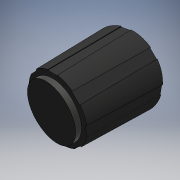
# Autodesk Inventor part: Knob-K60-S150
Saved by Autodesk Inventor 2018 (Build 220112000, 112)
## iProperties
Created: 2020-04-22
Part Number: Knob-K60-S150
Material: Všeobecné
Document SubType Name: Modeling
Designer: Jozko Mrkvicka
Density: 1 g/cm^3
Appearance: Výchozí
Author: Jozko Mrkvicka
Autodesk Inventor part; units mm, degrees
ref_plane "YZ Plane" through (0, 0, 0) normal (1, 0, 0) x (0, 1, 0)
ref_plane "XZ Plane" through (0, 0, 0) normal (0, 1, 0) x (-1, 0, 0)
ref_plane "XY Plane" through (0, 0, 0) normal (0, 0, 1) x (1, 0, 0)
sketch "Náčrt7" plane through (0, 0, 0) normal (0, 1, 0) x (-1, 0, 0)
  line L0 (7.4412, 0.9375) -> (7.3039, 0.9375)
  line L1 (7.3039, 0.9375) -> (7.3039, -0.9375)
  line L2 (7.3039, -0.9375) -> (7.4412, -0.9375)
  line L3 (-7.4412, -0.9375) -> (-7.3039, -0.9375)
  line L4 (-7.3039, -0.9375) -> (-7.3039, 0.9375)
  line L5 (-7.3039, 0.9375) -> (-7.4412, 0.9375)
  line L6 (-0.9375, 7.4412) -> (-0.9375, 7.3039)
  line L7 (-0.9375, 7.3039) -> (0.9375, 7.3039)
  line L8 (0.9375, 7.3039) -> (0.9375, 7.4412)
  line L9 (0.9375, -7.4412) -> (0.9375, -7.3039)
  line L10 (0.9375, -7.3039) -> (-0.9375, -7.3039)
  line L11 (-0.9375, -7.3039) -> (-0.9375, -7.4412)
  line L12 (-4.5988, -5.9246) -> (-4.5017, -5.8276)
  line L13 (-4.5017, -5.8276) -> (-5.8276, -4.5017)
  line L14 (-5.8276, -4.5017) -> (-5.9246, -4.5988)
  line L15 (4.5988, 5.9246) -> (4.5017, 5.8276)
  line L16 (4.5017, 5.8276) -> (5.8276, 4.5017)
  line L17 (5.8276, 4.5017) -> (5.9246, 4.5988)
  line L18 (5.9246, -4.5988) -> (5.8276, -4.5017)
  line L19 (5.8276, -4.5017) -> (4.5017, -5.8276)
  line L20 (4.5017, -5.8276) -> (4.6432, -5.969)
  line L21 (-5.9246, 4.5988) -> (-5.8276, 4.5017)
  line L22 (-5.8276, 4.5017) -> (-4.5017, 5.8276)
  line L23 (-4.5017, 5.8276) -> (-4.5988, 5.9246)
  arc A0 (5.9246, -4.5988) -> (7.4412, -0.9375) centre (0, 0) ccw
  arc A1 (0.9375, -7.4412) -> (4.5988, -5.9246) centre (0, 0) ccw
  arc A2 (-4.5988, -5.9246) -> (-0.9375, -7.4412) centre (0, 0) ccw
  arc A3 (-7.4412, -0.9375) -> (-5.9246, -4.5988) centre (0, 0) ccw
  arc A4 (-5.9246, 4.5988) -> (-7.4412, 0.9375) centre (0, 0) ccw
  arc A5 (-0.9375, 7.4412) -> (-4.5988, 5.9246) centre (0, 0) ccw
  arc A6 (7.4412, 0.9375) -> (5.9246, 4.5988) centre (0, 0) ccw
  arc A7 (4.5988, 5.9246) -> (0.9375, 7.4412) centre (0, 0) ccw
  point P0 (8, 0)
  point P1 (5.6569, -5.6569)
  point P2 (0, -8)
  point P3 (-5.6569, -5.6569)
  point P4 (-8, 0)
  point P5 (-5.6569, 5.6569)
  point P6 (0.0625, 7.5039)
  point P7 (5.6569, 5.6569)
  dimension "d237" = 0.2
  dimension "d239" = 7.5
  dimension "d240" = 7.5
  dimension "d241" = 7.5
  dimension "d242" = 7.5
  dimension "d243" = 7.5
  dimension "d244" = 7.5
  dimension "d245" = 7.5
  dimension "d246" = 7.5
  constraints: 48 end point, 16 point on circle, 8 centre point, 8 parallel, 8 perpendicular, 1 coincident, 1 horizontal, 1 point on line
  measures "d237" distance from line of L7 point (0.062, 7.504)
  measures "d239" radius of A7
  measures "d240" radius of A5
  measures "d241" radius of A4
  measures "d242" radius of A3
  measures "d243" radius of A2
  measures "d244" radius of A1
  measures "d245" radius of A0
  measures "d246" radius of A6
extrude "Vysunutí5" add sketch "Náčrt7" along normal blind 14
chamfer "Zkosení37" distance 1.5 distance2 14 1 edges at (-5.1647, 0, 5.1647) measured on face at (0.3125, 0, -1.4504)
chamfer "Zkosení38" distance 1.5 distance2 14 1 edges at (-7.3039, 0, 0) measured on face at (0.224, 0, -3.23)
chamfer "Zkosení39" distance 1.5 distance2 14 1 edges at (-6.9291, 0, 2.8701) measured on face at (-0.6473, 0, 0.9641)
chamfer "Zkosení40" distance 1.5 distance2 14 1 edges at (0, 0, 7.3039) measured on face at (-0.6473, 0, 0.9641)
chamfer "Zkosení41" distance 1.5 distance2 14 1 edges at (5.1647, 0, 5.1647) measured on face at (-0.1217, 0, -0.3202)
chamfer "Zkosení42" distance 1.5 distance2 14 1 edges at (7.3039, 0, 0) measured on face at (1.1549, 0, -1.1079)
chamfer "Zkosení43" distance 1.5 distance2 14 1 edges at (5.1647, 0, -5.1647) measured on face at (0.3125, 0, 1.3098)
chamfer "Zkosení44" distance 1.5 distance2 14 1 edges at (0, 0, -7.3039) measured on face at (-0.4752, 0, 0.0332)
chamfer "Zkosení45" distance 1.5 distance2 14 1 edges at (-5.1647, 0, -5.1647) measured on face at (-0.4752, 0, 0.0332)
chamfer "Zkosení46" distance 1.5 distance2 14 1 edges at (2.8701, 0, -6.9291) measured on face at (0.3125, 0, -1.2434)
chamfer "Zkosení47" distance 1.5 distance2 14 1 edges at (-6.9291, 0, -2.8701) measured on face at (0.3125, 0, -1.2434)
chamfer "Zkosení48" distance 1.5 distance2 14 1 edges at (-2.8701, 0, -6.9291) measured on face at (0.3125, 0, -1.2434)
chamfer "Zkosení49" distance 1.5 distance2 14 1 edges at (6.9291, 0, -2.8701) measured on face at (0.3125, 0, -1.2434)
chamfer "Zkosení50" distance 1.5 distance2 14 1 edges at (6.9291, 0, 2.8701) measured on face at (0.3125, 0, -1.2434)
chamfer "Zkosení51" distance 1.5 distance2 14 1 edges at (2.8701, 0, 6.9291) measured on face at (-0.4752, 0, 0.0332)
chamfer "Zkosení52" distance 1.5 distance2 14 1 edges at (-2.8701, 0, 6.9291) measured on face at (-0.4752, 0, 0.6582)
sketch "Náčrt8" plane through (0, 0, 0) normal (0, -1, 0) x (1, 0, 0)
  arc A0 (3.5276, 4.8534) -> (0.9375, 5.9263) centre (0, 0) ccw projected
  circle A1 centre (0, 0) radius 5
  dimension "d209" = 10
  constraints: 1 centre point, 1 coincident
  measures "d209" diameter of A1
extrude "Vysunutí6" add sketch "Náčrt8" along normal blind 1
sketch "Náčrt9" plane through (0, 14, 0) normal (0, 1, 0) x (1, 0, 0)
  arc A0 (-5.9246, 4.5988) -> (-7.4412, 0.9375) centre (0, 0) ccw projected
  circle A1 centre (0, 0) radius 6.75
  dimension "d247" = 13.5
  constraints: 1 centre point, 1 coincident
  measures "d247" diameter of A1
extrude "Vysunutí7" cut sketch "Náčrt9" against normal blind 0.1
sketch "Náčrt10" plane through (0, 13.9, 0) normal (0, 1, 0) x (1, 0, 0)
  circle A0 centre (0, 0) radius 6.75 projected
  circle A1 centre (0, 0) radius 5
  circle A2 centre (0, 0) radius 5.5
  point P0 (0, 5)
  dimension "d218" = 10
  dimension "d219" = 11
  constraints: 2 coincident, 1 centre point, 1 vertical alignment, 2 other
  measures "d219" diameter of A2
extrude "Vysunutí8" cut sketch "Náčrt10" against normal blind 1 contours A2
sketch "Náčrt11" plane through (0, 13.9, 0) normal (0, 1, 0) x (1, 0, 0)
  circle A0 centre (0, 0) radius 5 projected
  line L0 (0, 5.3) -> (-0.235, 4.9945)
  line L1 (0.235, 4.9945) -> (0, 5.3)
  line L2 (-0.235, 4.9945) -> (0.235, 4.9945)
  constraints: 6 end point, 2 point on circle
extrude "Vysunutí9" add sketch "Náčrt11" against normal blind 1 contours A0 L0 L1
pattern_circular "Kruhové pole1" count 60 over 360 about axis through (0, -10, 0) along (0, 1, 0) of "Vysunutí9"
sketch "Náčrt12" plane through (0, 13.9, 0) normal (0, 1, 0) x (1, 0, 0)
  arc A0 (-0.235, 4.9945) -> (0.235, 4.9945) centre (0, 0) ccw projected
  circle A1 centre (0, 0) radius 3
  point P0 (0.2883, 4.9917)
  dimension "d228" = 6
  constraints: 1 centre point, 1 coincident
  measures "d228" diameter of A1
extrude "Vysunutí10" add sketch "Náčrt12" along normal blind 0.1
sketch "Náčrt13" plane through (0, 14, 0) normal (0, 1, 0) x (1, 0, 0)
  circle A0 centre (0, 0) radius 3 projected
  line L0 (0.25, 1.9843) -> (0.25, 2.9896)
  line L1 (-0.25, 2.9896) -> (-0.25, 1.9843)
  line L2 (0.25, -2.9896) -> (0.25, -1.9843)
  line L3 (-0.25, -1.9843) -> (-0.25, -2.9896)
  line L4 (-1.9843, 0.25) -> (-2.9896, 0.25)
  line L5 (-3, -0.25) -> (-1.9843, -0.25)
  line L6 (2.9896, 0.25) -> (1.9843, 0.25)
  line L7 (1.9843, -0.25) -> (2.9896, -0.25)
  arc A1 (1.9843, 0.25) -> (0.25, 1.9843) centre (0, 0) ccw
  arc A2 (-0.25, 1.9843) -> (-1.9843, 0.25) centre (0, 0) ccw
  arc A3 (-1.9843, -0.25) -> (-0.25, -1.9843) centre (0, 0) ccw
  arc A4 (0.25, -1.9843) -> (1.9843, -0.25) centre (0, 0) ccw
  arc A5 (0.25, 2.9896) -> (-0.25, 2.9896) centre (0, 0) ccw
  arc A6 (2.9896, -0.25) -> (2.9896, 0.25) centre (0, 0) ccw
  arc A7 (-2.9896, 0.25) -> (-2.9896, -0.25) centre (0, 0) ccw
  arc A8 (-0.25, -2.9896) -> (0.25, -2.9896) centre (0, 0) ccw
  point P0 (0, 2.0559)
  point P1 (0, -2)
  point P2 (-2, 0)
  point P3 (2, 0)
  constraints: 16 end point, 16 point on circle, 8 centre point, 4 parallel, 2 coincident, 1 point on line
extrude "Vysunutí11" cut sketch "Náčrt13" against normal blind 7 contours A0 L7 A4 L2 L3 A3 L5 L4 A2 L1 L0 A1 L6
